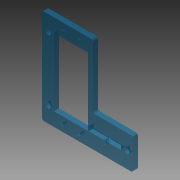
# Autodesk Inventor part: BracketCoxa
Saved by Autodesk Inventor 2015 (Build 190159000, 159)
## iProperties
Created: 2015-10-08
Part Number: BracketCoxa
Material: Generic
Document SubType Name: Modeling
Designer: styku
Density: 1 g/cm^3
Appearance: Clear
Author: styku
Autodesk Inventor part; units mm, degrees
ref_plane "YZ Plane" through (0, 0, 0) normal (1, 0, 0) x (0, 1, 0)
ref_plane "XZ Plane" through (0, 0, 0) normal (0, 1, 0) x (-1, 0, 0)
ref_plane "XY Plane" through (0, 0, 0) normal (0, 0, 1) x (1, 0, 0)
sketch "Sketch1" plane through (0, 0, 0) normal (0, 1, 0) x (-1, 0, 0)
  line L0 (46, 0) -> (-35, 0) construction
  line L1 (0, 54) -> (0, -60) construction
  line L2 (10, 20) -> (-10, 20)
  line L3 (-10, 20) -> (-10, -20)
  line L4 (-10, -20) -> (10, -20)
  line L5 (10, -20) -> (10, 20)
  line L6 (17, -28) -> (17, 28)
  line L7 (17, 28) -> (-13, 28)
  line L8 (-13, 28) -> (-13, -9.5)
  line L9 (-13, -9.5) -> (-36.5, -9.5)
  line L10 (-36.5, -9.5) -> (-36.5, -28)
  line L11 (-36.5, -28) -> (17, -28)
  line L12 (-29.5, -20) -> (-29.5, -17.5)
  line L13 (-10.5, -17.5) -> (-10.5, -20)
  circle A0 centre (5, 24.25) radius 0.5
  circle A1 centre (-5, 24.25) radius 0.5
  line L14 (14.6784, 24.25) -> (-18, 24.25) construction
  circle A2 centre (5, -24.25) radius 0.5
  circle A3 centre (-5, -24.25) radius 0.5
  circle A4 centre (13.5, -18.75) radius 1.5
  circle A5 centre (13.5, 18.75) radius 1.5
  circle A6 centre (-33, -18.75) radius 1.5
  line L15 (-20, 4) -> (-20, -26.5) construction
  line L16 (-10.5, -20) -> (-19.5, -20)
  line L17 (-19.5, -20) -> (-19.5, -22)
  line L18 (-19.5, -22) -> (-20.5, -22)
  line L19 (-20.5, -22) -> (-20.5, -20)
  line L20 (-20.5, -20) -> (-29.5, -20)
  line L21 (-10.5, -17.5) -> (-29.5, -17.5)
  point P0 (0, 0)
  point P1 (-20.5, -17.5)
  dimension "d0" = 40
  dimension "d1" = 20
  dimension "d2" = 7
  dimension "d3" = 8
  dimension "d4" = 8
  dimension "d5" = 3
  dimension "d6" = 20
  dimension "d7" = 10
  dimension "d8" = 19
  dimension "d9" = 2.5
  dimension "d10" = 0.5
  dimension "d11" = 1
  dimension "d12" = 1
  dimension "d13" = 5
  dimension "d14" = 5
  dimension "d15" = 4.25
  dimension "d16" = 3
  dimension "d17" = 9.25
  dimension "d19" = 18.5
  dimension "d20" = 7
  dimension "d21" = 3
  dimension "d23" = 9.25
  dimension "d29" = 3.5
  dimension "d30" = 3.5
  dimension "d31" = 2
  dimension "d32" = 1
  constraints: 44 end point, 13 perpendicular, 7 centre point, 4 horizontal, 3 parallel, 3 symmetric about line, 3 vertical, 2 collinear, 2 point on line, 5 other
  measures "d0" distance between parallel lines of L4 L2
  measures "d1" distance between parallel lines of L3 L5
  measures "d2" distance between parallel lines of L5 L6
  measures "d3" distance between parallel lines of L2 L7
  measures "d4" distance between parallel lines of L11 L4
  measures "d5" distance between parallel lines of L3 L8
  measures "d6" distance between parallel lines of L0 L2
  measures "d7" distance between parallel lines of L1 L5
  measures "d8" distance of L12.end L13.start
  measures "d9" distance of L12.start L12.end
  measures "d10" distance between parallel lines of L3 L13
  measures "d11" diameter of A1
  measures "d12" diameter of A0
  measures "d13" distance from line of A0.centre L5
  measures "d14" distance from line of L3 A1.centre
  measures "d15" distance between parallel lines of L2 L14
  measures "d16" diameter of A4
  measures "d17" distance from line of L11 A4.centre
  measures "d19" distance between parallel lines of L11 L9
  measures "d20" distance between parallel lines of L12 L10
  measures "d21" diameter of A6
  measures "d23" distance from line of L11 A6.centre
  measures "d29" distance from line of L5 A4.centre
  measures "d30" distance from line of A6.centre L12
  measures "d31" distance of L16.end L17.end
  measures "d32" distance of L17.end L18.end
extrude "Extrusion1" add sketch "Sketch1" along normal blind 3
fillet "Fillet1" radius 1 6 edges at (-17, 1.5, 28) (13, 1.5, 28) (13, 1.5, -9.5) (36.5, 1.5, -9.5) (36.5, 1.5, -28) (-17, 1.5, -28)
body "Solid1"
